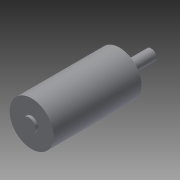
# Autodesk Inventor part: motor_43dsd
Saved by Autodesk Inventor 2013 (Build 170138000, 138)
## iProperties
Created: 2013-03-18
Part Number: motor_43dsd
Material: Generic
Document SubType Name: Modeling
Designer: Mahisorn
Density: 1 g/cm^3
Author: Mahisorn
Autodesk Inventor part; units mm, degrees
ref_plane "YZ Plane" through (0, 0, 0) normal (1, 0, 0) x (0, 1, 0)
ref_plane "XZ Plane" through (0, 0, 0) normal (0, 1, 0) x (-1, 0, 0)
ref_plane "XY Plane" through (0, 0, 0) normal (0, 0, 1) x (1, 0, 0)
sketch "Sketch1" plane through (0, 0, 0) normal (0, 1, 0) x (-1, 0, 0)
  circle A0 centre (0, 0) radius 8
  dimension "d0" = 16
  constraints: 1 centre point, 1 coincident
  measures "d0" diameter of A0
extrude "Extrusion1" add sketch "Sketch1" along normal blind 32
sketch "Sketch2" plane through (0, 32, 0) normal (0, 1, 0) x (1, 0, 0)
  circle A0 centre (0, 0) radius 8 projected
  circle A1 centre (0, 0) radius 3
  point P0 (5.5, 0)
  point P1 (-5.5, 0)
  dimension "d3" = 6
  dimension "d4" = 5.5
  dimension "d7" = 360
  constraints: 1 centre point, 1 coincident, 3 other
  measures "d3" diameter of A1
  measures "d4" distance of point (5.5, 0) A1.centre
extrude "Extrusion2" add sketch "Sketch2" along normal blind 1.5 contours A1
hole "Hole1" at (5.5, 32, 0) at (-5.5, 32, 0) direction (0, -1, 0) diameter 1.567 depth 3 tip angle 118 thread size "M2x0.4" class "6H" standard "ANSI Metric M Profile"
sketch "Sketch3" plane through (0, 33.5, 0) normal (0, 1, 0) x (1, 0, 0)
  circle A0 centre (0, 0) radius 3 projected
  circle A1 centre (0, 0) radius 2
  dimension "d18" = 4
  constraints: 1 centre point, 1 coincident
  measures "d18" diameter of A1
extrude "Extrusion3" add sketch "Sketch3" along normal blind 10 contours A1
sketch "Sketch4" plane through (0, 43.5, 0) normal (0, 1, 0) x (1, 0, 0)
  circle A0 centre (0, 0) radius 2 projected
  arc A1 (1.7321, 1) -> (-1.7321, 1) centre (0, 0) ccw
  line L0 (-1.7321, 1) -> (1.7321, 1)
  dimension "d21" = 1
  dimension "d23" = 1
  constraints: 2 end point, 2 point on circle, 1 centre point, 1 coincident, 3 other
  measures "d21" vertical distance of A1.centre L0.start
  measures "d23" vertical distance of point (0, 0) L0.end
extrude "Extrusion4" cut sketch "Sketch4" against normal blind 7.5 contours L0 A0 picked at (0.4849, 1.1242)
sketch "Sketch5" plane through (0, 0, 0) normal (0, -1, 0) x (1, 0, 0)
  circle A0 centre (0, 0) radius 8 projected
  circle A1 centre (0, 0) radius 2.5
  dimension "d26" = 5
  constraints: 1 centre point, 1 coincident
  measures "d26" diameter of A1
extrude "Extrusion5" add sketch "Sketch5" along normal blind 1 contours A1
body "Solid1"
